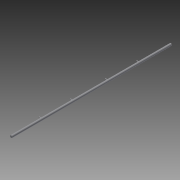
# Autodesk Inventor part: X_Rail-Rod-Rev1
Saved by Autodesk Inventor 2015 (Build 190159000, 159)
## iProperties
Created: 2016-12-21
Part Number: X_Rail-Rod-Rev1
Material: Generic
Document SubType Name: Modeling
Designer: Guy
Density: 1 g/cm^3
Appearance: Default
Author: Guy
Autodesk Inventor part; units mm, degrees
ref_plane "YZ Plane" through (0, 0, 0) normal (1, 0, 0) x (0, 1, 0)
ref_plane "XZ Plane" through (0, 0, 0) normal (0, 1, 0) x (-1, 0, 0)
ref_plane "XY Plane" through (0, 0, 0) normal (0, 0, 1) x (1, 0, 0)
sketch "Sketch1" plane through (0, 0, 0) normal (0, 1, 0) x (-1, 0, 0)
  circle A0 centre (0, 0) radius 15
  dimension "d0" = 30
  constraints: 1 centre point, 1 coincident
  measures "d0" diameter of A0
extrude "Extrusion1" add sketch "Sketch1" along normal blind 2050
sketch "Sketch2" plane through (0, 0, 0) normal (0, -1, 0) x (1, 0, 0)
  circle A0 centre (0, 0) radius 15 projected
  line L0 (0, 15) -> (0, -15)
  constraints: 2 end point, 2 point on circle, 1 vertical
extrude "Extrusion2" add sketch "Sketch2" along normal blind 0.1 contours A0 L0 picked at (3.1174, 3.9092)
sketch "Sketch4" plane through (0, 0, 0) normal (1, 0, 0) x (0, 1, 0)
  line L0 (2050, -15) -> (2050, 15) projected
  line L1 (0, 15) -> (0, -15) projected
  line L2 (0, 15) -> (-0.1, 15) projected
  line L3 (-0.1, -15) -> (-0.1, 15) projected
  line L4 (0, -15) -> (-0.1, -15) projected
  line L5 (-0.1, 15) -> (2050, 15) projected
  line L6 (-0.1, -15) -> (2050, -15) projected
  circle A0 centre (400, 0) radius 5
  circle A1 centre (800, 0) radius 5
  circle A2 centre (1250, 0) radius 5
  circle A3 centre (1650, 0) radius 5
  line L7 (1025, 15) -> (1025, -15)
  point P0 (0, 0)
  dimension "d9" = 1025
  dimension "d10" = 400
  dimension "d11" = 400
  dimension "d12" = 400
  dimension "d13" = 400
  dimension "d14" = 10
  dimension "d15" = 10
  dimension "d16" = 10
  dimension "d17" = 10
  constraints: 4 centre point, 2 end point, 2 point on line, 1 perpendicular
  measures "d9" distance between parallel lines of L0 L7
  measures "d10" distance from line of A3.centre L0
  measures "d11" distance of A2.centre A3.centre
  measures "d12" distance from line of A0.centre L1
  measures "d13" distance of A1.centre A0.centre
  measures "d14" diameter of A0
  measures "d15" diameter of A1
  measures "d16" diameter of A2
  measures "d17" diameter of A3
extrude "Extrusion3" add sketch "Sketch4" against normal blind 40 contours A0 | A1 | A2 | A3
body "Solid1"
